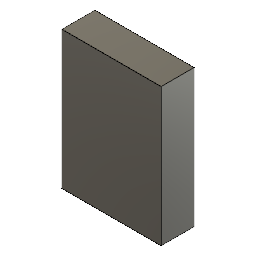
TAPA v2 (Autodesk Fusion 360 design; units mm, degrees)
Autodesk Fusion 360 part; units mm, degrees
sketch "Boceto1" plane through (0, 0, 0) normal (0, 1, 0) x (1, 0, 0)
  line L0 (58, 0) -> (62, 0)
  line L1 (62, 0) -> (62, -4)
  line L2 (62, -4) -> (58, -4)
  line L3 (58, -4) -> (58, 0)
  line L4 (58, -8) -> (62, -8)
  line L5 (62, -8) -> (62, -12)
  line L6 (62, -12) -> (58, -12)
  line L7 (58, -12) -> (58, -8)
  line L8 (62, -12) -> (62, -21)
  line L9 (62, -21) -> (-4, -21)
  line L10 (62, 0) -> (65, 0)
  line L11 (65, 0) -> (65, -24)
  line L12 (65, -24) -> (-7, -24)
  line L13 (29, -21) -> (29, -3)
  line L14 (-4, -12) -> (0, -12)
  line L15 (0, -8) -> (-4, -8)
  line L16 (-4, -8) -> (-4, -12)
  line L17 (-4, -12) -> (-4, -21)
  line L18 (-4, -4) -> (0, -4)
  line L19 (-4, 0) -> (-4, -4)
  line L20 (-4, 0) -> (-7, 0)
  line L21 (-7, 0) -> (-7, -24)
  line L22 (-7, -24) -> (65, -24)
  line L23 (-4, -21) -> (62, -21)
  line L24 (0, 0) -> (-4, 0)
  line L25 (-4, -4) -> (-4, -8)
  line L26 (62, -8) -> (62, -4)
  line L27 (0, -16) -> (0, -8)
  line L28 (0, -4) -> (0, 0)
  line L29 (58, 0) -> (58, -4)
  line L30 (58, -8) -> (58, -16)
  dimension "d1" = 58
  dimension "d2" = 16
  dimension "d3" = 4
  dimension "d4" = 4
  dimension "d5" = 4
  dimension "d6" = 4
  dimension "d7" = 4
  dimension "d8" = 9
  dimension "d9" = 66
  dimension "d10" = 24
  dimension "d11" = 72
  constraint vertical L29
  constraint vertical L27
  constraint coincident L24.start L28.end
  constraint horizontal L0
  constraint vertical L1
  constraint horizontal L2
  constraint vertical L3
  constraint horizontal L4
  constraint vertical L5
  constraint horizontal L6
  constraint vertical L7
  constraint perpendicular L6 L8
  constraint perpendicular L8 L9
  constraint perpendicular L1 L10
  constraint perpendicular L9 L11
  constraint perpendicular L8 L12
  constraint midpoint L9 L13.start
  constraint perpendicular L9 L13
  constraint symmetric L0.start L13 L24.start
  constraint symmetric L0.end L13 L19.start
  constraint symmetric L1.end L13 L18.start
  constraint symmetric L2.end L13 L18.end
  constraint symmetric L4.start L13 L15.start
  constraint symmetric L4.end L13 L15.end
  constraint symmetric L5.end L13 L14.start
  constraint symmetric L6.end L13 L14.end
  constraint symmetric L8.end L13 L9.end
  constraint symmetric L9.end L13 L8.end
  constraint symmetric L10.end L13 L20.end
  constraint symmetric L11.end L13 L12.end
  constraint symmetric L12.end L13 L11.end
  constraint collinear L27 L28
  constraint collinear L29 L30
  measures "d1" distance of L24.start L0.start
  measures "d2" distance of L24.start L27.start
  measures "d3" distance of L0.start L0.end
  measures "d4" distance of L0.start L2.end
  measures "d5" distance of L2.end L4.start
  measures "d6" distance of L4.start L4.end
  measures "d7" distance of L4.start L6.end
  measures "d8" distance of L5.end L8.end
  measures "d9" distance of L8.end L9.end
  measures "d10" distance of L10.end L11.end
  measures "d11" distance of L11.end L12.end
extrude "Extruir1" add sketch "Boceto1" along normal blind 100
sketch "Boceto2" plane through (0, 100, 0) normal (0, 1, 0) x (-1, 0, 0)
  line L0 (-62, 8) -> (-58, 8)
  line L1 (-58, 8) -> (-58, 12)
  line L2 (-58, 12) -> (-62, 12)
  line L3 (-62, 12) -> (-62, 21)
  line L4 (-62, 21) -> (4, 21)
  line L5 (4, 21) -> (4, 12)
  line L6 (4, 12) -> (0, 12)
  line L7 (0, 12) -> (0, 8)
  line L8 (0, 8) -> (4, 8)
  line L9 (4, 8) -> (4, 4)
  line L10 (4, 4) -> (0, 4)
  line L11 (0, 4) -> (0, 0)
  line L12 (0, 0) -> (7, 0)
  line L13 (7, 0) -> (7, 24)
  line L14 (7, 24) -> (-65, 24)
  line L15 (-65, 24) -> (-65, 0)
  line L16 (-65, 0) -> (-58, 0)
  line L17 (-58, 0) -> (-58, 4)
  line L18 (-58, 4) -> (-62, 4)
  line L19 (-62, 4) -> (-62, 8)
  line L20 (7, 0) -> (-65, 0)
  line L21 (-65, 0) -> (-65, 24)
  line L22 (-65, 24) -> (7, 24)
  line L23 (7, 24) -> (7, 0)
  constraint horizontal L20
  constraint vertical L21
  constraint horizontal L22
  constraint vertical L23
  constraint coincident L14.end L15.start
  constraint coincident L12.end L13.start
extrude "Extruir2" add sketch "Boceto2" against normal blind 3 contours L0 L1 L2 L3 L4 L5 L6 L7 L8 L9 L10 L11 L17 L18 L19 L20
move_face "CarasDesfase1" offset -0.2 14 faces at (58, 32.3333, 2.6667) (58, 32.3333, 10.6667) (62, 32.3333, 15) (59.3333, 32.3333, 8) (62, 32.3333, 6.6667) (0, 32.3333, 2.6667) (-4, 32.3333, 5.3333) (0, 32.3333, 10.6667) (-4, 32.3333, 15) (-1.3333, 32.3333, 8) (-2.6667, 32.3333, 4) (-2.6667, 32.3333, 12) (59.3333, 64.6667, 4) (59.3333, 64.6667, 12)
